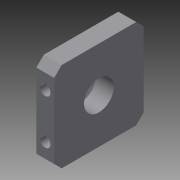
# Autodesk Inventor part: 1.5 in bearing block
Saved by Autodesk Inventor 2015 (Build 190159000, 159)
## iProperties
Created: 2015-01-21
Part Number: 1.5 in bearing block
Material: Generic
Document SubType Name: Modeling
Designer: chapale16
Density: 1 g/cm^3
Appearance: Default
Author: chapale16
Autodesk Inventor part; units mm, degrees
ref_plane "YZ Plane" through (0, 0, 0) normal (1, 0, 0) x (0, 1, 0)
ref_plane "XZ Plane" through (0, 0, 0) normal (0, 1, 0) x (-1, 0, 0)
ref_plane "XY Plane" through (0, 0, 0) normal (0, 0, 1) x (1, 0, 0)
sketch "Sketch1" plane through (0, 0, 0) normal (1, 0, 0) x (0, 1, 0)
  line L0 (0, 0) -> (38.1, 0)
  line L1 (38.1, 0) -> (38.1, -38.1)
  line L2 (38.1, -38.1) -> (0, -38.1)
  line L3 (0, -38.1) -> (0, 0)
  circle A0 centre (19.05, -19.05) radius 6.35
  dimension "d0" = 38.1
  dimension "d1" = 38.1
  dimension "d2" = 12.7
  constraints: 8 end point, 2 parallel, 1 centre point, 1 horizontal, 1 perpendicular
  measures "d0" distance of L1.end L2.end
  measures "d1" distance of L0.end L1.end
  measures "d2" diameter of A0
extrude "Extrusion1" add sketch "Sketch1" along normal blind 7.62
chamfer "Chamfer1" distance 3.175 angle 45 4 edges at (3.81, 38.1, 0) (3.81, 38.1, -38.1) (3.81, 0, 0) (3.81, 0, -38.1)
sketch "Sketch2" plane through (0, 3.175, -38.1) normal (0, 0, -1) x (-1, 0, 0)
  line L0 (0, 0) -> (-7.62, 0) projected
  line L1 (0, 31.75) -> (0, 0) projected
  line L2 (-7.62, 31.75) -> (0, 31.75) projected
  line L3 (-7.62, 0) -> (-7.62, 31.75) projected
  line L4 (-3.81, 15.875) -> (-3.81, 25.4)
  line L5 (-3.81, 25.4) -> (-3.81, 6.35)
  point P0 (0, -3.175)
  dimension "d10" = 9.525
  dimension "d11" = 19.05
  constraints: 4 end point, 2 coincident, 1 point on line, 1 vertical
  measures "d10" distance of L4.start L4.end
  measures "d11" distance of L4.end L5.end
hole "Hole1" at (3.81, 28.575, -38.1) at (3.81, 9.525, -38.1) direction (0, 0, 1) diameter 4.445 end through all
body "Solid1"
